Autodesk Fusion 360 part; units mm, degrees
(part 6 of 8)
  spline S1138 degree 3 poles (86.7419, -11.2934) (84.8369, -11.1346) (82.5615, -11.2934) (81.6884, -11.2934) knots 0 0 0 0 1 1 1 1
  spline S1139 degree 3 poles (81.6884, -11.2934) (80.7359, -11.2934) (80.5771, -11.0817) (80.3125, -10.6584) knots 0 0 0 0 1 1 1 1
  line L266 (80.3125, -10.6584) -> (72.6925, 1.486)
  line L267 (72.6925, 1.486) -> (72.6925, -8.9121)
  spline S1140 degree 3 poles (72.6925, -8.9121) (72.6925, -10.0498) (74.28, -9.9705) (74.28, -10.3938) knots 0 0 0 0 1 1 1 1
  spline S1141 degree 3 poles (74.28, -10.3938) (74.28, -10.7113) (73.989, -11.2934) (73.7773, -11.2669) knots 0 0 0 0 1 1 1 1
  spline S1142 degree 3 poles (73.7773, -11.2669) (73.3805, -11.214) (72.6132, -11.1902) (71.8459, -11.1902) knots 0 0 0 0 1 1 1 1
  spline S1143 degree 3 poles (71.8459, -11.1902) (71.0786, -11.1902) (70.2848, -11.214) (69.888, -11.2669) knots 0 0 0 0 1 1 1 1
  spline S1144 degree 3 poles (69.888, -11.2669) (69.6763, -11.2934) (69.4117, -10.7113) (69.4117, -10.3938) knots 0 0 0 0 1 1 1 1
  spline S1145 degree 3 poles (69.4117, -10.3938) (69.4117, -9.9705) (70.7082, -10.0498) (70.7082, -8.9121) knots 0 0 0 0 1 1 1 1
  spline S1146 degree 3 poles (250.4624, -9.4413) (247.4194, -9.4413) (245.779, -7.0865) (245.779, -2.4034) knots -1 -1 -1 -1 0 0 0 0
  spline S1147 degree 3 poles (252.1822, -8.8328) (252.1822, -9.4942) (251.7853, -9.4413) (250.4624, -9.4413) knots -1 -1 -1 -1 0 0 0 0
  line L268 (252.1822, -8.8328) -> (252.1822, 4.026)
  spline S1148 degree 3 poles (250.4357, 4.6345) (250.8328, 4.6345) (252.1822, 4.6875) (252.1822, 4.026) knots -1 -1 -1 -1 0 0 0 0
  spline S1149 degree 3 poles (245.779, -2.4034) (245.779, 2.2797) (247.4194, 4.6345) (250.4357, 4.6345) knots -1 -1 -1 -1 0 0 0 0
  spline S1150 degree 3 poles (239.9579, -2.3769) (239.9579, 2.9677) (243.6621, 6.5131) (249.245, 6.5131) knots 0 0 0 0 1 1 1 1
  spline S1151 degree 3 poles (249.245, 6.5131) (252.0234, 6.4866) (253.1082, 6.4337) (254.9606, 6.4337) knots 0 0 0 0 1 1 1 1
  spline S1152 degree 3 poles (254.9606, 6.4337) (256.1247, 6.4337) (257.4212, 6.4602) (258.4795, 6.5131) knots 0 0 0 0 1 1 1 1
  spline S1153 degree 3 poles (258.4795, 6.5131) (258.6912, 6.5131) (258.9558, 5.9575) (258.9558, 5.64) knots 0 0 0 0 1 1 1 1
  spline S1154 degree 3 poles (258.9558, 5.64) (258.9558, 5.2166) (257.527, 5.296) (257.527, 4.1583) knots 0 0 0 0 1 1 1 1
  line L269 (257.527, 4.1583) -> (257.527, -8.965)
  spline S1155 degree 3 poles (257.527, -8.965) (257.527, -10.0763) (258.9825, -9.9969) (258.9825, -10.4203) knots 0 0 0 0 1 1 1 1
  spline S1156 degree 3 poles (258.9825, -10.4203) (258.9825, -10.7378) (258.6912, -11.3225) (258.4795, -11.2934) knots 0 0 0 0 1 1 1 1
  spline S1157 degree 3 poles (258.4795, -11.2934) (257.4212, -11.2405) (256.1512, -11.214) (254.9606, -11.214) knots 0 0 0 0 1 1 1 1
  spline S1158 degree 3 poles (254.9606, -11.214) (253.1082, -11.214) (252.0234, -11.2934) (249.245, -11.2934) knots 0 0 0 0 1 1 1 1
  spline S1159 degree 3 poles (249.245, -11.2934) (243.6885, -11.2934) (239.9579, -7.7215) (239.9579, -2.3769) knots 0 0 0 0 1 1 1 1
  line L270 (70.7082, 2.0681) -> (70.7082, -8.9121)
  line L271 (70.7082, -8.9121) -> (70.7082, 2.0681)
  spline S1160 degree 3 poles (72.6925, -8.9121) (72.6925, -10.0498) (74.28, -9.9705) (74.28, -10.3938) knots 0 0 0 0 1 1 1 1
  spline S1161 degree 3 poles (74.28, -10.3938) (74.28, -9.9705) (72.6925, -10.0498) (72.6925, -8.9121) knots -1 -1 -1 -1 0 0 0 0
  spline S1162 degree 3 poles (239.9579, -2.3769) (239.9579, 2.9677) (243.6621, 6.5131) (249.245, 6.5131) knots 0 0 0 0 1 1 1 1
  spline S1163 degree 3 poles (249.245, 6.5131) (243.6621, 6.5131) (239.9579, 2.9677) (239.9579, -2.3769) knots -1 -1 -1 -1 0 0 0 0
  line L272 (83.9373, -6.2928) -> (76.2909, 5.9045)
  line L273 (76.2909, 5.9045) -> (83.9373, -6.2928)
  spline S1164 degree 3 poles (-114.9509, -10.3938) (-114.9509, -9.9705) (-113.7604, -9.9972) (-113.3886, -8.9388) knots 0 0 0 0 1 1 1 1
  spline S1165 degree 3 poles (-113.3886, -8.9388) (-113.7604, -9.9972) (-114.9509, -9.9705) (-114.9509, -10.3938) knots -1 -1 -1 -1 0 0 0 0
  line L274 (257.527, -8.965) -> (257.527, 4.1583)
  line L275 (257.527, 4.1583) -> (257.527, -8.965)
  line L276 (72.6925, -8.9121) -> (72.6925, 1.486)
  line L277 (72.6925, 1.486) -> (72.6925, -8.9121)
  spline S1166 degree 3 poles (254.9606, 6.4337) (256.1247, 6.4337) (257.4212, 6.4602) (258.4795, 6.5131) knots 0 0 0 0 1 1 1 1
  spline S1167 degree 3 poles (258.4795, 6.5131) (257.4212, 6.4602) (256.1247, 6.4337) (254.9606, 6.4337) knots -1 -1 -1 -1 0 0 0 0
  spline S1168 degree 3 poles (-91.5045, -10.3938) (-91.5045, -9.9705) (-89.8408, -9.9972) (-90.2088, -8.9388) knots 0 0 0 0 1 1 1 1
  spline S1169 degree 3 poles (-90.2088, -8.9388) (-89.8408, -9.9972) (-91.5045, -9.9705) (-91.5045, -10.3938) knots -1 -1 -1 -1 0 0 0 0
  line L278 (83.9373, 4.1583) -> (83.9373, -6.2928)
  line L279 (83.9373, -6.2928) -> (83.9373, 4.1583)
  spline S1170 degree 3 poles (258.9558, 5.64) (258.9558, 5.2166) (257.527, 5.296) (257.527, 4.1583) knots 0 0 0 0 1 1 1 1
  spline S1171 degree 3 poles (257.527, 4.1583) (257.527, 5.296) (258.9558, 5.2166) (258.9558, 5.64) knots -1 -1 -1 -1 0 0 0 0
  line L280 (72.6925, 1.486) -> (80.3125, -10.6584)
  line L281 (80.3125, -10.6584) -> (72.6925, 1.486)
  spline S1172 degree 3 poles (249.245, -11.2934) (243.6885, -11.2934) (239.9579, -7.7215) (239.9579, -2.3769) knots 0 0 0 0 1 1 1 1
  spline S1173 degree 3 poles (239.9579, -2.3769) (239.9579, -7.7215) (243.6885, -11.2934) (249.245, -11.2934) knots -1 -1 -1 -1 0 0 0 0
  spline S1174 degree 3 poles (120.1059, -10.4203) (120.1059, -10.0234) (121.5611, -10.1028) (121.5611, -8.965) knots 0 0 0 0 1 1 1 1
  line L282 (121.5611, -8.965) -> (121.5611, 3.7085)
  spline S1175 degree 3 poles (121.5611, 3.7085) (121.5611, 4.3964) (121.27, 4.5552) (119.6296, 4.5552) knots 0 0 0 0 1 1 1 1
  spline S1176 degree 3 poles (119.6296, 4.5552) (115.7667, 4.5552) (114.7348, 1.486) (114.2321, 1.486) knots 0 0 0 0 1 1 1 1
  spline S1177 degree 3 poles (114.2321, 1.486) (113.9146, 1.486) (113.3325, 1.7506) (113.3325, 1.9622) knots 0 0 0 0 1 1 1 1
  spline S1178 degree 3 poles (113.3325, 1.9622) (113.3325, 2.1739) (114.0469, 5.3489) (114.1527, 5.7458) knots 0 0 0 0 1 1 1 1
  spline S1179 degree 3 poles (114.1527, 5.7458) (114.338, 6.3543) (114.5496, 6.5395) (115.1052, 6.5131) knots 0 0 0 0 1 1 1 1
  spline S1180 degree 3 poles (115.1052, 6.5131) (116.9573, 6.4602) (119.2063, 6.4337) (121.4552, 6.4337) knots 0 0 0 0 1 1 1 1
  spline S1181 degree 3 poles (121.4552, 6.4337) (123.7307, 6.4337) (125.9796, 6.4602) (127.8317, 6.5131) knots 0 0 0 0 1 1 1 1
  spline S1182 degree 3 poles (127.8317, 6.5131) (128.0698, 6.5131) (128.3344, 5.9575) (128.3344, 5.64) knots 0 0 0 0 1 1 1 1
  spline S1183 degree 3 poles (128.3344, 5.64) (128.3344, 5.2166) (126.9057, 5.296) (126.9057, 4.1847) knots 0 0 0 0 1 1 1 1
  line L283 (126.9057, 4.1847) -> (126.9057, -8.965)
  spline S1184 degree 3 poles (126.9057, -8.965) (126.9057, -10.1028) (128.3344, -9.9969) (128.3344, -10.4203) knots 0 0 0 0 1 1 1 1
  spline S1185 degree 3 poles (128.3344, -10.4203) (128.3344, -10.7378) (128.0698, -11.3225) (127.8317, -11.2934) knots 0 0 0 0 1 1 1 1
  spline S1186 degree 3 poles (127.8317, -11.2934) (126.7734, -11.2405) (125.5034, -11.214) (124.2069, -11.214) knots 0 0 0 0 1 1 1 1
  spline S1187 degree 3 poles (124.2069, -11.214) (122.9369, -11.214) (121.6405, -11.2405) (120.6086, -11.2934) knots 0 0 0 0 1 1 1 1
  spline S1188 degree 3 poles (120.6086, -11.2934) (120.3969, -11.3225) (120.1059, -10.7378) (120.1059, -10.4203) knots 0 0 0 0 1 1 1 1
  spline S1189 degree 3 poles (-125.2401, 5.64) (-125.2401, 5.2164) (-127.0384, 5.1106) (-126.4299, 4.1584) knots 0 0 0 0 1 1 1 1
  spline S1190 degree 3 poles (-126.4299, 4.1584) (-127.0384, 5.1106) (-125.2401, 5.2164) (-125.2401, 5.64) knots -1 -1 -1 -1 0 0 0 0
  spline S1191 degree 3 poles (120.1059, -10.4203) (120.1059, -10.0234) (121.5611, -10.1028) (121.5611, -8.965) knots 0 0 0 0 1 1 1 1
  spline S1192 degree 3 poles (121.5611, -8.965) (121.5611, -10.1028) (120.1059, -10.0234) (120.1059, -10.4203) knots -1 -1 -1 -1 0 0 0 0
  spline S1193 degree 3 poles (121.5611, -8.965) (121.5611, -10.1028) (120.1059, -10.0234) (120.1059, -10.4203) knots -1 -1 -1 -1 0 0 0 0
  spline S1194 degree 3 poles (120.1059, -10.4203) (120.1059, -10.7378) (120.3969, -11.3225) (120.6086, -11.2934) knots -1 -1 -1 -1 0 0 0 0
  spline S1195 degree 3 poles (120.6086, -11.2934) (121.6405, -11.2405) (122.9369, -11.214) (124.2069, -11.214) knots -1 -1 -1 -1 0 0 0 0
  spline S1196 degree 3 poles (124.2069, -11.214) (125.5034, -11.214) (126.7734, -11.2405) (127.8317, -11.2934) knots -1 -1 -1 -1 0 0 0 0
  spline S1197 degree 3 poles (127.8317, -11.2934) (128.0698, -11.3225) (128.3344, -10.7378) (128.3344, -10.4203) knots -1 -1 -1 -1 0 0 0 0
  spline S1198 degree 3 poles (128.3344, -10.4203) (128.3344, -9.9969) (126.9057, -10.1028) (126.9057, -8.965) knots -1 -1 -1 -1 0 0 0 0
  line L284 (126.9057, -8.965) -> (126.9057, 4.1847)
  spline S1199 degree 3 poles (126.9057, 4.1847) (126.9057, 5.296) (128.3344, 5.2166) (128.3344, 5.64) knots -1 -1 -1 -1 0 0 0 0
  spline S1200 degree 3 poles (128.3344, 5.64) (128.3344, 5.9575) (128.0698, 6.5131) (127.8317, 6.5131) knots -1 -1 -1 -1 0 0 0 0
  spline S1201 degree 3 poles (127.8317, 6.5131) (125.9796, 6.4602) (123.7307, 6.4337) (121.4552, 6.4337) knots -1 -1 -1 -1 0 0 0 0
  spline S1202 degree 3 poles (121.4552, 6.4337) (119.2063, 6.4337) (116.9573, 6.4602) (115.1052, 6.5131) knots -1 -1 -1 -1 0 0 0 0
  spline S1203 degree 3 poles (115.1052, 6.5131) (114.5496, 6.5395) (114.338, 6.3543) (114.1527, 5.7458) knots -1 -1 -1 -1 0 0 0 0
  spline S1204 degree 3 poles (114.1527, 5.7458) (114.0469, 5.3489) (113.3325, 2.1739) (113.3325, 1.9622) knots -1 -1 -1 -1 0 0 0 0
  spline S1205 degree 3 poles (113.3325, 1.9622) (113.3325, 1.7506) (113.9146, 1.486) (114.2321, 1.486) knots -1 -1 -1 -1 0 0 0 0
  spline S1206 degree 3 poles (114.2321, 1.486) (114.7348, 1.486) (115.7667, 4.5552) (119.6296, 4.5552) knots -1 -1 -1 -1 0 0 0 0
  spline S1207 degree 3 poles (119.6296, 4.5552) (121.27, 4.5552) (121.5611, 4.3964) (121.5611, 3.7085) knots -1 -1 -1 -1 0 0 0 0
  line L285 (121.5611, 3.7085) -> (121.5611, -8.965)
  spline S1208 degree 3 poles (250.4624, -9.4413) (247.4194, -9.4413) (245.779, -7.0865) (245.779, -2.4034) knots -1 -1 -1 -1 0 0 0 0
  spline S1209 degree 3 poles (250.4624, -9.4413) (247.4194, -9.4413) (245.779, -7.0865) (245.779, -2.4034) knots -1 -1 -1 -1 0 0 0 0
  spline S1210 degree 3 poles (250.4624, -9.4413) (247.4194, -9.4413) (245.779, -7.0865) (245.779, -2.4034) knots -1 -1 -1 -1 0 0 0 0
  spline S1211 degree 3 poles (245.779, -2.4034) (245.779, 2.2797) (247.4194, 4.6345) (250.4357, 4.6345) knots -1 -1 -1 -1 0 0 0 0
  spline S1212 degree 3 poles (250.4357, 4.6345) (250.8328, 4.6345) (252.1822, 4.6875) (252.1822, 4.026) knots -1 -1 -1 -1 0 0 0 0
  line L286 (252.1822, 4.026) -> (252.1822, -8.8328)
  spline S1213 degree 3 poles (252.1822, -8.8328) (252.1822, -9.4942) (251.7853, -9.4413) (250.4624, -9.4413) knots -1 -1 -1 -1 0 0 0 0
  spline S1214 degree 3 poles (249.245, 6.5131) (243.6621, 6.5131) (239.9579, 2.9677) (239.9579, -2.3769) knots -1 -1 -1 -1 0 0 0 0
  spline S1215 degree 3 poles (239.9579, -2.3769) (239.9579, -7.7215) (243.6885, -11.2934) (249.245, -11.2934) knots -1 -1 -1 -1 0 0 0 0
  spline S1216 degree 3 poles (249.245, -11.2934) (252.0234, -11.2934) (253.1082, -11.214) (254.9606, -11.214) knots -1 -1 -1 -1 0 0 0 0
  spline S1217 degree 3 poles (254.9606, -11.214) (256.1512, -11.214) (257.4212, -11.2405) (258.4795, -11.2934) knots -1 -1 -1 -1 0 0 0 0
  spline S1218 degree 3 poles (258.4795, -11.2934) (258.6912, -11.3225) (258.9825, -10.7378) (258.9825, -10.4203) knots -1 -1 -1 -1 0 0 0 0
  spline S1219 degree 3 poles (258.9825, -10.4203) (258.9825, -9.9969) (257.527, -10.0763) (257.527, -8.965) knots -1 -1 -1 -1 0 0 0 0
  line L287 (257.527, -8.965) -> (257.527, 4.1583)
  spline S1220 degree 3 poles (257.527, 4.1583) (257.527, 5.296) (258.9558, 5.2166) (258.9558, 5.64) knots -1 -1 -1 -1 0 0 0 0
  spline S1221 degree 3 poles (258.9558, 5.64) (258.9558, 5.9575) (258.6912, 6.5131) (258.4795, 6.5131) knots -1 -1 -1 -1 0 0 0 0
  spline S1222 degree 3 poles (258.4795, 6.5131) (257.4212, 6.4602) (256.1247, 6.4337) (254.9606, 6.4337) knots -1 -1 -1 -1 0 0 0 0
  spline S1223 degree 3 poles (254.9606, 6.4337) (253.1082, 6.4337) (252.0234, 6.4866) (249.245, 6.5131) knots -1 -1 -1 -1 0 0 0 0
  spline S1224 degree 3 poles (263.4264, -11.0288) (262.765, -11.0288) (262.5533, -11.2934) (262.1297, -11.2934) knots 0 0 0 0 1 1 1 1
  spline S1225 degree 3 poles (262.1297, -11.2934) (262.5533, -11.2934) (262.765, -11.0288) (263.4264, -11.0288) knots -1 -1 -1 -1 0 0 0 0
  spline S1226 degree 3 poles (276.4447, -2.3769) (276.4447, -7.748) (272.6876, -11.558) (267.4219, -11.558) knots 0 0 0 0 1 1 1 1
  spline S1227 degree 3 poles (267.4219, -11.558) (272.6876, -11.558) (276.4447, -7.748) (276.4447, -2.3769) knots -1 -1 -1 -1 0 0 0 0
  spline S1228 degree 3 poles (266.6546, -9.653) (269.1417, -9.653) (270.6236, -7.2717) (270.6236, -3.303) knots 0 0 0 0 1 1 1 1
  spline S1229 degree 3 poles (270.6236, -3.303) (270.6236, -7.2717) (269.1417, -9.653) (266.6546, -9.653) knots -1 -1 -1 -1 0 0 0 0
  spline S1230 degree 3 poles (-167.8359, 5.746) (-167.6766, 6.3543) (-167.4397, 6.5397) (-166.9127, 6.5132) knots 0 0 0 0 1 1 1 1
  spline S1231 degree 3 poles (-166.9127, 6.5132) (-167.4397, 6.5397) (-167.6766, 6.3543) (-167.8359, 5.746) knots -1 -1 -1 -1 0 0 0 0
  spline S1232 degree 3 poles (-153.918, -6.1339) (-153.5994, -6.1339) (-153.0438, -6.4252) (-153.0438, -6.6368) knots 0 0 0 0 1 1 1 1
  spline S1233 degree 3 poles (-153.0438, -6.6368) (-153.0438, -6.4252) (-153.5994, -6.1339) (-153.918, -6.1339) knots -1 -1 -1 -1 0 0 0 0
  spline S1234 degree 3 poles (-154.6329, -11.2934) (-158.334, -11.2138) (-163.9224, -11.1901) (-167.6235, -11.2934) knots 0 0 0 0 1 1 1 1
  spline S1235 degree 3 poles (-167.6235, -11.2934) (-163.9224, -11.1901) (-158.334, -11.2138) (-154.6329, -11.2934) knots -1 -1 -1 -1 0 0 0 0
  spline S1236 degree 3 poles (68.1959, -2.3768) (68.1959, -7.8007) (64.3845, -11.5577) (58.909, -11.5577) knots 0 0 0 0 1 1 1 1
  spline S1237 degree 3 poles (58.909, -11.5577) (64.3845, -11.5577) (68.1959, -7.8007) (68.1959, -2.3768) knots -1 -1 -1 -1 0 0 0 0
  spline S1238 degree 3 poles (49.6221, -2.3768) (49.6221, 3.0471) (53.406, 6.7777) (58.909, 6.7777) knots 0 0 0 0 1 1 1 1
  spline S1239 degree 3 poles (58.909, 6.7777) (53.406, 6.7777) (49.6221, 3.0471) (49.6221, -2.3768) knots -1 -1 -1 -1 0 0 0 0
  spline S1240 degree 3 poles (-120.4768, 5.6133) (-120.4768, 5.9311) (-120.1048, 6.5396) (-119.8955, 6.5132) knots 0 0 0 0 1 1 1 1
  spline S1241 degree 3 poles (-119.8955, 6.5132) (-120.1048, 6.5396) (-120.4768, 5.9311) (-120.4768, 5.6133) knots -1 -1 -1 -1 0 0 0 0
  spline S1242 degree 3 poles (55.4435, -2.3768) (55.4435, 2.5179) (56.5282, 4.9256) (58.909, 4.9256) knots -1 -1 -1 -1 0 0 0 0
  spline S1243 degree 3 poles (58.909, -9.7058) (56.5529, -9.7058) (55.4435, -7.3509) (55.4435, -2.3768) knots -1 -1 -1 -1 0 0 0 0
  spline S1244 degree 3 poles (62.3744, -2.3768) (62.3744, -7.2715) (61.2897, -9.7058) (58.909, -9.7058) knots -1 -1 -1 -1 0 0 0 0
  spline S1245 degree 3 poles (58.909, 4.9256) (61.2897, 4.9256) (62.3744, 2.5179) (62.3744, -2.3768) knots -1 -1 -1 -1 0 0 0 0
  spline S1246 degree 3 poles (68.1959, -2.3768) (68.1959, -7.8007) (64.3845, -11.5577) (58.909, -11.5577) knots 0 0 0 0 1 1 1 1
  spline S1247 degree 3 poles (58.909, -11.5577) (53.4307, -11.5577) (49.6221, -7.8007) (49.6221, -2.3768) knots 0 0 0 0 1 1 1 1
  spline S1248 degree 3 poles (49.6221, -2.3768) (49.6221, 3.0471) (53.406, 6.7777) (58.909, 6.7777) knots 0 0 0 0 1 1 1 1
  spline S1249 degree 3 poles (58.909, 6.7777) (64.4119, 6.7777) (68.1959, 3.0471) (68.1959, -2.3768) knots 0 0 0 0 1 1 1 1
  spline S1250 degree 3 poles (55.4435, -2.3768) (55.4435, 2.5179) (56.5282, 4.9256) (58.909, 4.9256) knots -1 -1 -1 -1 0 0 0 0
  spline S1251 degree 3 poles (58.909, 4.9256) (61.2897, 4.9256) (62.3744, 2.5179) (62.3744, -2.3768) knots -1 -1 -1 -1 0 0 0 0
  spline S1252 degree 3 poles (62.3744, -2.3768) (62.3744, -7.2715) (61.2897, -9.7058) (58.909, -9.7058) knots -1 -1 -1 -1 0 0 0 0
  spline S1253 degree 3 poles (58.909, -9.7058) (56.5529, -9.7058) (55.4435, -7.3509) (55.4435, -2.3768) knots -1 -1 -1 -1 0 0 0 0
  spline S1254 degree 3 poles (58.909, -11.5577) (64.3845, -11.5577) (68.1959, -7.8007) (68.1959, -2.3768) knots -1 -1 -1 -1 0 0 0 0
  spline S1255 degree 3 poles (68.1959, -2.3768) (68.1959, 3.0471) (64.4119, 6.7777) (58.909, 6.7777) knots -1 -1 -1 -1 0 0 0 0
  spline S1256 degree 3 poles (58.909, 6.7777) (53.406, 6.7777) (49.6221, 3.0471) (49.6221, -2.3768) knots -1 -1 -1 -1 0 0 0 0
  spline S1257 degree 3 poles (49.6221, -2.3768) (49.6221, -7.8007) (53.4307, -11.5577) (58.909, -11.5577) knots -1 -1 -1 -1 0 0 0 0
  spline S1258 degree 3 poles (58.909, -9.7058) (56.5529, -9.7058) (55.4435, -7.3509) (55.4435, -2.3768) knots -1 -1 -1 -1 0 0 0 0
  spline S1259 degree 3 poles (58.909, -9.7058) (56.5529, -9.7058) (55.4435, -7.3509) (55.4435, -2.3768) knots -1 -1 -1 -1 0 0 0 0
  spline S1260 degree 3 poles (58.909, -11.5577) (53.4307, -11.5577) (49.6221, -7.8007) (49.6221, -2.3768) knots 0 0 0 0 1 1 1 1
  spline S1261 degree 3 poles (49.6221, -2.3768) (49.6221, -7.8007) (53.4307, -11.5577) (58.909, -11.5577) knots -1 -1 -1 -1 0 0 0 0
  spline S1262 degree 3 poles (-159.9516, 3.7083) (-159.6044, 4.2905) (-160.2417, 4.5552) (-161.5939, 4.5552) knots 0 0 0 0 1 1 1 1
  spline S1263 degree 3 poles (-161.5939, 4.5552) (-160.2417, 4.5552) (-159.6044, 4.2905) (-159.9516, 3.7083) knots -1 -1 -1 -1 0 0 0 0
  line L288 (151.9352, 6.2485) -> (151.9352, -8.9386)
  spline S1264 degree 3 poles (151.9352, -8.9386) (151.9352, -10.0763) (150.48, -9.9969) (150.48, -10.3938) knots -1 -1 -1 -1 0 0 0 0
  spline S1265 degree 3 poles (150.48, -10.3938) (150.48, -10.7113) (150.7684, -11.2934) (150.9827, -11.2934) knots -1 -1 -1 -1 0 0 0 0
  spline S1266 degree 3 poles (150.9827, -11.2934) (152.012, -11.2405) (153.3111, -11.214) (154.6075, -11.214) knots -1 -1 -1 -1 0 0 0 0
  spline S1267 degree 3 poles (154.6075, -11.214) (155.8775, -11.214) (157.174, -11.2405) (158.2323, -11.2934) knots -1 -1 -1 -1 0 0 0 0
  spline S1268 degree 3 poles (158.2323, -11.2934) (158.444, -11.2934) (158.7086, -10.7113) (158.7086, -10.3938) knots -1 -1 -1 -1 0 0 0 0
  spline S1269 degree 3 poles (158.7086, -10.3938) (158.7086, -9.9969) (157.2798, -10.0763) (157.2798, -8.9386) knots -1 -1 -1 -1 0 0 0 0
  line L289 (157.2798, -8.9386) -> (157.2798, 6.4866)
  spline S1270 degree 3 poles (157.2798, 6.4866) (157.2798, 9.6881) (158.4175, 10.6141) (161.0634, 10.6141) knots -1 -1 -1 -1 0 0 0 0
  spline S1271 degree 3 poles (161.0634, 10.6141) (161.3015, 10.6141) (161.7248, 11.5931) (161.5661, 11.7518) knots -1 -1 -1 -1 0 0 0 0
  spline S1272 degree 3 poles (161.5661, 11.7518) (161.2221, 12.0958) (159.7669, 12.5985) (157.7825, 12.5985) knots -1 -1 -1 -1 0 0 0 0
  spline S1273 degree 3 poles (157.7825, 12.5985) (153.8932, 12.5985) (151.9352, 10.5612) (151.9352, 6.2485) knots -1 -1 -1 -1 0 0 0 0
  line L290 (-84.4965, -8.9388) -> (-89.9196, 6.5129)
  line L291 (-89.9196, 6.5129) -> (-94.7607, 6.5129)
  spline S1274 degree 3 poles (-94.7607, 6.5129) (-95.2114, 3.9993) (-97.7765, -0.8688) (-99.0459, -5.0229) knots -1 -1 -1 -1 0 0 0 0
  line L292 (-99.0459, -5.0229) -> (-103.0944, 6.5129)
  spline S1275 degree 3 poles (-103.0944, 6.5129) (-104.0221, 6.46) (-104.7619, 6.4337) (-105.5281, 6.4337) knots -1 -1 -1 -1 0 0 0 0
  spline S1276 degree 3 poles (-105.5281, 6.4337) (-106.2717, 6.4337) (-107.0378, 6.46) (-107.9354, 6.5129) knots -1 -1 -1 -1 0 0 0 0
  line L293 (-107.9354, 6.5129) -> (-113.3886, -8.9388)
  spline S1277 degree 3 poles (-113.3886, -8.9388) (-113.7604, -9.9972) (-114.9509, -9.9705) (-114.9509, -10.3938) knots -1 -1 -1 -1 0 0 0 0
  spline S1278 degree 3 poles (-114.9509, -10.3938) (-114.9509, -10.7115) (-114.688, -11.2936) (-114.4439, -11.267) knots -1 -1 -1 -1 0 0 0 0
  spline S1279 degree 3 poles (-114.4439, -11.267) (-114.0496, -11.214) (-113.2534, -11.1903) (-112.4609, -11.1903) knots -1 -1 -1 -1 0 0 0 0
  spline S1280 degree 3 poles (-112.4609, -11.1903) (-111.6685, -11.1903) (-110.8723, -11.214) (-110.478, -11.267) knots -1 -1 -1 -1 0 0 0 0
  spline S1281 degree 3 poles (-110.478, -11.267) (-110.2639, -11.2936) (-109.9747, -10.7115) (-109.9747, -10.3938) knots -1 -1 -1 -1 0 0 0 0
  spline S1282 degree 3 poles (-109.9747, -10.3938) (-109.9747, -9.9705) (-111.6422, -9.9972) (-111.2704, -8.9122) knots -1 -1 -1 -1 0 0 0 0
  line L294 (-111.2704, -8.9122) -> (-107.327, 2.4384)
  line L295 (-107.327, 2.4384) -> (-103.3873, -8.9122)
  spline S1283 degree 3 poles (-103.3873, -8.9122) (-103.0155, -9.9972) (-104.7093, -9.9705) (-104.7093, -10.3938) knots -1 -1 -1 -1 0 0 0 0
  spline S1284 degree 3 poles (-104.7093, -10.3938) (-104.7093, -10.7115) (-104.4163, -11.267) (-104.206, -11.267) knots -1 -1 -1 -1 0 0 0 0
  spline S1285 degree 3 poles (-104.206, -11.267) (-103.1733, -11.214) (-101.7987, -11.1903) (-100.3978, -11.1903) knots -1 -1 -1 -1 0 0 0 0
  spline S1286 degree 3 poles (-100.3978, -11.1903) (-99.0195, -11.1903) (-97.645, -11.214) (-96.5859, -11.267) knots -1 -1 -1 -1 0 0 0 0
  spline S1287 degree 3 poles (-96.5859, -11.267) (-96.3755, -11.267) (-96.1089, -10.7115) (-96.1089, -10.3938) knots -1 -1 -1 -1 0 0 0 0
  spline S1288 degree 3 poles (-96.1089, -10.3938) (-96.1089, -9.9705) (-97.2994, -9.9972) (-97.6712, -8.9388) knots -1 -1 -1 -1 0 0 0 0
  spline S1289 degree 3 poles (-97.6712, -8.9388) (-98.1219, -7.0866) (-95.3165, -1.2924) (-94.0996, 2.2533) knots -1 -1 -1 -1 0 0 0 0
  line L296 (-94.0996, 2.2533) -> (-90.2088, -8.9388)
  spline S1290 degree 3 poles (-90.2088, -8.9388) (-89.8408, -9.9972) (-91.5045, -9.9705) (-91.5045, -10.3938) knots -1 -1 -1 -1 0 0 0 0
  spline S1291 degree 3 poles (-91.5045, -10.3938) (-91.5045, -10.7115) (-91.2416, -11.267) (-91.0313, -11.267) knots -1 -1 -1 -1 0 0 0 0
  spline S1292 degree 3 poles (-91.0313, -11.267) (-89.9722, -11.214) (-88.5939, -11.1903) (-87.2194, -11.1903) knots -1 -1 -1 -1 0 0 0 0
  spline S1293 degree 3 poles (-87.2194, -11.1903) (-85.8448, -11.1903) (-84.4664, -11.214) (-83.4111, -11.267) knots -1 -1 -1 -1 0 0 0 0
  spline S1294 degree 3 poles (-83.4111, -11.267) (-83.1971, -11.267) (-82.9079, -10.7115) (-82.9079, -10.3938) knots -1 -1 -1 -1 0 0 0 0
  spline S1295 degree 3 poles (-82.9079, -10.3938) (-82.9079, -9.9705) (-84.1247, -9.9972) (-84.4965, -8.9388) knots -1 -1 -1 -1 0 0 0 0
  spline S1296 degree 3 poles (158.7086, -10.3938) (158.7086, -10.7113) (158.444, -11.2934) (158.2323, -11.2934) knots 0 0 0 0 1 1 1 1
  spline S1297 degree 3 poles (158.2323, -11.2934) (158.444, -11.2934) (158.7086, -10.7113) (158.7086, -10.3938) knots -1 -1 -1 -1 0 0 0 0
  spline S1298 degree 3 poles (-153.2807, 6.5132) (-153.0438, 6.5132) (-152.7783, 5.9576) (-152.7783, 5.6398) knots 0 0 0 0 1 1 1 1
  spline S1299 degree 3 poles (-152.7783, 5.6398) (-152.7783, 5.9576) (-153.0438, 6.5132) (-153.2807, 6.5132) knots -1 -1 -1 -1 0 0 0 0
  spline S1300 degree 3 poles (82.3498, 5.6135) (82.3498, 5.931) (82.6409, 6.5395) (82.8525, 6.5131) knots 0 0 0 0 1 1 1 1
  spline S1301 degree 3 poles (82.8525, 6.5131) (82.6409, 6.5395) (82.3498, 5.931) (82.3498, 5.6135) knots -1 -1 -1 -1 0 0 0 0
  spline S1302 degree 3 poles (86.7419, -11.2934) (84.8369, -11.1346) (82.5615, -11.2934) (81.6884, -11.2934) knots 0 0 0 0 1 1 1 1
  spline S1303 degree 3 poles (81.6884, -11.2934) (82.5615, -11.2934) (84.8369, -11.1346) (86.7419, -11.2934) knots -1 -1 -1 -1 0 0 0 0
  spline S1304 degree 3 poles (226.6509, 0.507) (226.6509, 0.7187) (227.233, 1.0097) (227.5505, 1.0097) knots 0 0 0 0 1 1 1 1
  spline S1305 degree 3 poles (227.5505, 1.0097) (227.233, 1.0097) (226.6509, 0.7187) (226.6509, 0.507) knots -1 -1 -1 -1 0 0 0 0
  spline S1306 degree 3 poles (237.5515, -8.9386) (237.5515, -10.0763) (238.9803, -9.9969) (238.9803, -10.3938) knots 0 0 0 0 1 1 1 1
  spline S1307 degree 3 poles (238.9803, -10.3938) (238.9803, -9.9969) (237.5515, -10.0763) (237.5515, -8.9386) knots -1 -1 -1 -1 0 0 0 0
  spline S1308 degree 3 poles (227.5505, 1.0097) (228.3443, 1.0097) (228.1855, -1.7155) (230.3551, -1.7684) knots 0 0 0 0 1 1 1 1
  spline S1309 degree 3 poles (230.3551, -1.7684) (228.1855, -1.7155) (228.3443, 1.0097) (227.5505, 1.0097) knots -1 -1 -1 -1 0 0 0 0
  line L297 (237.5515, -8.9386) -> (237.5515, 4.1847)
  line L298 (237.5515, 4.1847) -> (237.5515, -8.9386)
  line L299 (232.2072, -1.8213) -> (230.3551, -1.7684)
  line L300 (230.3551, -1.7684) -> (232.2072, -1.8213)
  spline S1310 degree 3 poles (-82.9079, -10.3938) (-82.9079, -10.7115) (-83.1971, -11.267) (-83.4111, -11.267) knots 0 0 0 0 1 1 1 1
  spline S1311 degree 3 poles (-83.4111, -11.267) (-83.1971, -11.267) (-82.9079, -10.7115) (-82.9079, -10.3938) knots -1 -1 -1 -1 0 0 0 0
  spline S1312 degree 3 poles (154.6075, -11.214) (153.3111, -11.214) (152.012, -11.2405) (150.9827, -11.2934) knots 0 0 0 0 1 1 1 1
  spline S1313 degree 3 poles (150.9827, -11.2934) (152.012, -11.2405) (153.3111, -11.214) (154.6075, -11.214) knots -1 -1 -1 -1 0 0 0 0
  spline S1314 degree 3 poles (-134.0225, 6.5132) (-132.9915, 6.4601) (-131.4296, 6.4338) (-129.8948, 6.4338) knots 0 0 0 0 1 1 1 1
  spline S1315 degree 3 poles (-129.8948, 6.4338) (-131.4296, 6.4338) (-132.9915, 6.4601) (-134.0225, 6.5132) knots -1 -1 -1 -1 0 0 0 0
  spline S1316 degree 3 poles (121.4552, 6.4337) (123.7307, 6.4337) (125.9796, 6.4602) (127.8317, 6.5131) knots 0 0 0 0 1 1 1 1
  spline S1317 degree 3 poles (127.8317, 6.5131) (125.9796, 6.4602) (123.7307, 6.4337) (121.4552, 6.4337) knots -1 -1 -1 -1 0 0 0 0
  spline S1318 degree 3 poles (124.2069, -11.214) (122.9369, -11.214) (121.6405, -11.2405) (120.6086, -11.2934) knots 0 0 0 0 1 1 1 1
  spline S1319 degree 3 poles (120.6086, -11.2934) (121.6405, -11.2405) (122.9369, -11.214) (124.2069, -11.214) knots -1 -1 -1 -1 0 0 0 0
  spline S1320 degree 3 poles (120.6086, -11.2934) (120.3969, -11.3225) (120.1059, -10.7378) (120.1059, -10.4203) knots 0 0 0 0 1 1 1 1
  spline S1321 degree 3 poles (120.1059, -10.4203) (120.1059, -10.7378) (120.3969, -11.3225) (120.6086, -11.2934) knots -1 -1 -1 -1 0 0 0 0
  spline S1322 degree 3 poles (223.3172, 1.9622) (223.3172, 2.1739) (224.0316, 5.3489) (224.1374, 5.7458) knots 0 0 0 0 1 1 1 1
  spline S1323 degree 3 poles (224.1374, 5.7458) (224.0316, 5.3489) (223.3172, 2.1739) (223.3172, 1.9622) knots -1 -1 -1 -1 0 0 0 0
  spline S1324 degree 3 poles (-166.9127, 6.5132) (-165.0581, 6.4601) (-162.5703, 6.4339) (-160.1069, 6.4339) knots 0 0 0 0 1 1 1 1
  spline S1325 degree 3 poles (-160.1069, 6.4339) (-162.5703, 6.4339) (-165.0581, 6.4601) (-166.9127, 6.5132) knots -1 -1 -1 -1 0 0 0 0
  spline S1326 degree 3 poles (161.0634, 10.6141) (158.4175, 10.6141) (157.2798, 9.6881) (157.2798, 6.4866) knots 0 0 0 0 1 1 1 1
  spline S1327 degree 3 poles (157.2798, 6.4866) (157.2798, 9.6881) (158.4175, 10.6141) (161.0634, 10.6141) knots -1 -1 -1 -1 0 0 0 0
  spline S1328 degree 3 poles (-168.657, 1.9624) (-168.657, 2.174) (-167.9421, 5.3489) (-167.8359, 5.746) knots 0 0 0 0 1 1 1 1
  spline S1329 degree 3 poles (-167.8359, 5.746) (-167.9421, 5.3489) (-168.657, 2.174) (-168.657, 1.9624) knots -1 -1 -1 -1 0 0 0 0
  spline S1330 degree 3 poles (157.2798, -8.9386) (157.2798, -10.0763) (158.7086, -9.9969) (158.7086, -10.3938) knots 0 0 0 0 1 1 1 1
  spline S1331 degree 3 poles (158.7086, -10.3938) (158.7086, -9.9969) (157.2798, -10.0763) (157.2798, -8.9386) knots -1 -1 -1 -1 0 0 0 0
  spline S1332 degree 3 poles (-153.0438, -6.6368) (-153.0438, -6.8484) (-153.6525, -10.1292) (-153.7301, -10.5524) knots 0 0 0 0 1 1 1 1
  spline S1333 degree 3 poles (-153.7301, -10.5524) (-153.6525, -10.1292) (-153.0438, -6.8484) (-153.0438, -6.6368) knots -1 -1 -1 -1 0 0 0 0
  spline S1334 degree 3 poles (-114.4439, -11.267) (-114.688, -11.2936) (-114.9509, -10.7115) (-114.9509, -10.3938) knots 0 0 0 0 1 1 1 1
  spline S1335 degree 3 poles (-114.9509, -10.3938) (-114.9509, -10.7115) (-114.688, -11.2936) (-114.4439, -11.267) knots -1 -1 -1 -1 0 0 0 0
  spline S1336 degree 3 poles (83.9373, 4.1583) (83.9373, 5.296) (82.3498, 5.2166) (82.3498, 5.6135) knots 0 0 0 0 1 1 1 1
  spline S1337 degree 3 poles (82.3498, 5.6135) (82.3498, 5.2166) (83.9373, 5.296) (83.9373, 4.1583) knots -1 -1 -1 -1 0 0 0 0
  line L301 (-94.0996, 2.2533) -> (-90.2088, -8.9388)
  line L302 (-90.2088, -8.9388) -> (-94.0996, 2.2533)
  spline S1338 degree 3 poles (81.6884, -11.2934) (80.7359, -11.2934) (80.5771, -11.0817) (80.3125, -10.6584) knots 0 0 0 0 1 1 1 1
  spline S1339 degree 3 poles (80.3125, -10.6584) (80.5771, -11.0817) (80.7359, -11.2934) (81.6884, -11.2934) knots -1 -1 -1 -1 0 0 0 0
  spline S1340 degree 3 poles (-112.4609, -11.1903) (-113.2534, -11.1903) (-114.0496, -11.214) (-114.4439, -11.267) knots 0 0 0 0 1 1 1 1
  spline S1341 degree 3 poles (-114.4439, -11.267) (-114.0496, -11.214) (-113.2534, -11.1903) (-112.4609, -11.1903) knots -1 -1 -1 -1 0 0 0 0
  spline S1342 degree 3 poles (223.6347, -10.6848) (223.6347, -10.1028) (224.0316, -6.9807) (224.0316, -6.769) knots 0 0 0 0 1 1 1 1
  spline S1343 degree 3 poles (224.0316, -6.769) (224.0316, -6.9807) (223.6347, -10.1028) (223.6347, -10.6848) knots -1 -1 -1 -1 0 0 0 0
  spline S1344 degree 3 poles (227.5505, -6.5044) (227.233, -6.5044) (226.6509, -6.2134) (226.6509, -6.0017) knots 0 0 0 0 1 1 1 1
  spline S1345 degree 3 poles (226.6509, -6.0017) (226.6509, -6.2134) (227.233, -6.5044) (227.5505, -6.5044) knots -1 -1 -1 -1 0 0 0 0
  spline S1346 degree 3 poles (238.4778, -11.2934) (236.7313, -11.2405) (234.3236, -11.214) (231.8897, -11.214) knots 0 0 0 0 1 1 1 1
  spline S1347 degree 3 poles (231.8897, -11.214) (234.3236, -11.214) (236.7313, -11.2405) (238.4778, -11.2934) knots -1 -1 -1 -1 0 0 0 0
  spline S1348 degree 3 poles (226.6509, -6.0017) (226.7832, -3.8321) (226.7832, -1.6625) (226.6509, 0.507) knots 0 0 0 0 1 1 1 1
  spline S1349 degree 3 poles (226.6509, 0.507) (226.7832, -1.6625) (226.7832, -3.8321) (226.6509, -6.0017) knots -1 -1 -1 -1 0 0 0 0
  spline S1350 degree 3 poles (238.9803, -10.3938) (238.9803, -10.7113) (238.7157, -11.2934) (238.4778, -11.2934) knots 0 0 0 0 1 1 1 1
  spline S1351 degree 3 poles (238.4778, -11.2934) (238.7157, -11.2934) (238.9803, -10.7113) (238.9803, -10.3938) knots -1 -1 -1 -1 0 0 0 0
  spline S1352 degree 3 poles (265.5433, 3.7879) (263.8233, 3.7879) (262.4475, 3.0206) (260.8862, 1.2743) knots 0 0 0 0 1 1 1 1
  spline S1353 degree 3 poles (260.8862, 1.2743) (262.4475, 3.0206) (263.8233, 3.7879) (265.5433, 3.7879) knots -1 -1 -1 -1 0 0 0 0
  spline S1354 degree 3 poles (270.6236, -3.303) (270.6236, 1.195) (268.7186, 3.7879) (265.5433, 3.7879) knots 0 0 0 0 1 1 1 1
  spline S1355 degree 3 poles (265.5433, 3.7879) (263.8233, 3.7879) (262.4475, 3.0206) (260.8862, 1.2743) knots 0 0 0 0 1 1 1 1
  spline S1356 degree 3 poles (260.8862, 1.2743) (260.7277, 1.0891) (259.9339, 1.3272) (259.9339, 1.5389) knots 0 0 0 0 1 1 1 1
  spline S1357 degree 3 poles (259.9339, 1.5389) (259.9339, 2.412) (262.2093, 6.7777) (267.66, 6.7777) knots 0 0 0 0 1 1 1 1
  spline S1358 degree 3 poles (267.66, 6.7777) (272.767, 6.7777) (276.4447, 2.9412) (276.4447, -2.3769) knots 0 0 0 0 1 1 1 1
  spline S1359 degree 3 poles (276.4447, -2.3769) (276.4447, -7.748) (272.6876, -11.558) (267.4219, -11.558) knots 0 0 0 0 1 1 1 1
  spline S1360 degree 3 poles (267.4219, -11.558) (265.305, -11.558) (264.326, -11.0288) (263.4264, -11.0288) knots 0 0 0 0 1 1 1 1
  spline S1361 degree 3 poles (263.4264, -11.0288) (262.765, -11.0288) (262.5533, -11.2934) (262.1297, -11.2934) knots 0 0 0 0 1 1 1 1
  spline S1362 degree 3 poles (262.1297, -11.2934) (261.786, -11.2934) (261.5743, -10.9759) (261.442, -10.4732) knots 0 0 0 0 1 1 1 1
  spline S1363 degree 3 poles (261.442, -10.4732) (261.336, -10.0763) (260.7539, -6.7161) (260.7539, -6.5044) knots 0 0 0 0 1 1 1 1
  spline S1364 degree 3 poles (260.7539, -6.5044) (260.7539, -6.2928) (261.336, -5.7371) (261.6537, -5.7371) knots 0 0 0 0 1 1 1 1
  spline S1365 degree 3 poles (261.6537, -5.7371) (262.1297, -5.7371) (263.4529, -9.653) (266.6546, -9.653) knots 0 0 0 0 1 1 1 1
  spline S1366 degree 3 poles (266.6546, -9.653) (269.1417, -9.653) (270.6236, -7.2717) (270.6236, -3.303) knots 0 0 0 0 1 1 1 1
  spline S1367 degree 3 poles (270.6236, -3.303) (270.6236, 1.195) (268.7186, 3.7879) (265.5433, 3.7879) knots 0 0 0 0 1 1 1 1
  spline S1368 degree 3 poles (265.5433, 3.7879) (268.7186, 3.7879) (270.6236, 1.195) (270.6236, -3.303) knots -1 -1 -1 -1 0 0 0 0
  line L303 (157.2798, -8.9386) -> (157.2798, 6.4866)
  line L304 (157.2798, 6.4866) -> (157.2798, -8.9386)
  spline S1369 degree 3 poles (-168.126, -10.42) (-168.126, -10.0234) (-168.1791, -9.9175) (-167.599, -8.9649) knots 0 0 0 0 1 1 1 1
  spline S1370 degree 3 poles (-167.599, -8.9649) (-168.1791, -9.9175) (-168.126, -10.0234) (-168.126, -10.42) knots -1 -1 -1 -1 0 0 0 0
  spline S1371 degree 3 poles (150.9827, -11.2934) (150.7684, -11.2934) (150.48, -10.7113) (150.48, -10.3938) knots 0 0 0 0 1 1 1 1
  spline S1372 degree 3 poles (150.48, -10.3938) (150.48, -10.7113) (150.7684, -11.2934) (150.9827, -11.2934) knots -1 -1 -1 -1 0 0 0 0
  line L305 (-89.9196, 6.5129) -> (-84.4965, -8.9388)
  spline S1373 degree 3 poles (-84.4965, -8.9388) (-84.1247, -9.9972) (-82.9079, -9.9705) (-82.9079, -10.3938) knots 0 0 0 0 1 1 1 1
  spline S1374 degree 3 poles (-82.9079, -10.3938) (-82.9079, -10.7115) (-83.1971, -11.267) (-83.4111, -11.267) knots 0 0 0 0 1 1 1 1
  spline S1375 degree 3 poles (-83.4111, -11.267) (-84.4664, -11.214) (-85.8448, -11.1903) (-87.2194, -11.1903) knots 0 0 0 0 1 1 1 1
  spline S1376 degree 3 poles (-87.2194, -11.1903) (-88.5939, -11.1903) (-89.9722, -11.214) (-91.0313, -11.267) knots 0 0 0 0 1 1 1 1
  spline S1377 degree 3 poles (-91.0313, -11.267) (-91.2416, -11.267) (-91.5045, -10.7115) (-91.5045, -10.3938) knots 0 0 0 0 1 1 1 1
  spline S1378 degree 3 poles (-91.5045, -10.3938) (-91.5045, -9.9705) (-89.8408, -9.9972) (-90.2088, -8.9388) knots 0 0 0 0 1 1 1 1
  line L306 (-90.2088, -8.9388) -> (-94.0996, 2.2533)
  spline S1379 degree 3 poles (-94.0996, 2.2533) (-95.3165, -1.2924) (-98.1219, -7.0866) (-97.6712, -8.9388) knots 0 0 0 0 1 1 1 1
  spline S1380 degree 3 poles (-97.6712, -8.9388) (-97.2994, -9.9972) (-96.1089, -9.9705) (-96.1089, -10.3938) knots 0 0 0 0 1 1 1 1
  spline S1381 degree 3 poles (-96.1089, -10.3938) (-96.1089, -10.7115) (-96.3755, -11.267) (-96.5859, -11.267) knots 0 0 0 0 1 1 1 1
  spline S1382 degree 3 poles (-96.5859, -11.267) (-97.645, -11.214) (-99.0195, -11.1903) (-100.3978, -11.1903) knots 0 0 0 0 1 1 1 1
  spline S1383 degree 3 poles (-100.3978, -11.1903) (-101.7987, -11.1903) (-103.1733, -11.214) (-104.206, -11.267) knots 0 0 0 0 1 1 1 1
  spline S1384 degree 3 poles (-104.206, -11.267) (-104.4163, -11.267) (-104.7093, -10.7115) (-104.7093, -10.3938) knots 0 0 0 0 1 1 1 1
  spline S1385 degree 3 poles (-104.7093, -10.3938) (-104.7093, -9.9705) (-103.0155, -9.9972) (-103.3873, -8.9122) knots 0 0 0 0 1 1 1 1
  line L307 (-103.3873, -8.9122) -> (-107.327, 2.4384)
  line L308 (-107.327, 2.4384) -> (-111.2704, -8.9122)
  spline S1386 degree 3 poles (-111.2704, -8.9122) (-111.6422, -9.9972) (-109.9747, -9.9705) (-109.9747, -10.3938) knots 0 0 0 0 1 1 1 1
  spline S1387 degree 3 poles (-109.9747, -10.3938) (-109.9747, -10.7115) (-110.2639, -11.2936) (-110.478, -11.267) knots 0 0 0 0 1 1 1 1
  spline S1388 degree 3 poles (-110.478, -11.267) (-110.8723, -11.214) (-111.6685, -11.1903) (-112.4609, -11.1903) knots 0 0 0 0 1 1 1 1
  spline S1389 degree 3 poles (-112.4609, -11.1903) (-113.2534, -11.1903) (-114.0496, -11.214) (-114.4439, -11.267) knots 0 0 0 0 1 1 1 1
  spline S1390 degree 3 poles (-114.4439, -11.267) (-114.688, -11.2936) (-114.9509, -10.7115) (-114.9509, -10.3938) knots 0 0 0 0 1 1 1 1
  spline S1391 degree 3 poles (-114.9509, -10.3938) (-114.9509, -9.9705) (-113.7604, -9.9972) (-113.3886, -8.9388) knots 0 0 0 0 1 1 1 1
  line L309 (-113.3886, -8.9388) -> (-107.9354, 6.5129)
  spline S1392 degree 3 poles (-107.9354, 6.5129) (-107.0378, 6.46) (-106.2717, 6.4337) (-105.5281, 6.4337) knots 0 0 0 0 1 1 1 1
  spline S1393 degree 3 poles (-105.5281, 6.4337) (-104.7619, 6.4337) (-104.0221, 6.46) (-103.0944, 6.5129) knots 0 0 0 0 1 1 1 1
  line L310 (-103.0944, 6.5129) -> (-99.0459, -5.0229)
  spline S1394 degree 3 poles (-99.0459, -5.0229) (-97.7765, -0.8688) (-95.2114, 3.9993) (-94.7607, 6.5129) knots 0 0 0 0 1 1 1 1
  line L311 (-94.7607, 6.5129) -> (-89.9196, 6.5129)
  spline S1395 degree 3 poles (151.9352, 6.2485) (151.9352, 10.5612) (153.8932, 12.5985) (157.7825, 12.5985) knots 0 0 0 0 1 1 1 1
  spline S1396 degree 3 poles (157.7825, 12.5985) (153.8932, 12.5985) (151.9352, 10.5612) (151.9352, 6.2485) knots -1 -1 -1 -1 0 0 0 0
  spline S1397 degree 3 poles (-159.8169, -9.362) (-155.8503, -9.362) (-154.4205, -6.1339) (-153.918, -6.1339) knots 0 0 0 0 1 1 1 1
  spline S1398 degree 3 poles (-153.918, -6.1339) (-154.4205, -6.1339) (-155.8503, -9.362) (-159.8169, -9.362) knots -1 -1 -1 -1 0 0 0 0
  line L312 (-159.9516, 3.7083) -> (-167.599, -8.9649)
  line L313 (-167.599, -8.9649) -> (-159.9516, 3.7083)
  line L314 (151.9352, -8.9386) -> (151.9352, 6.2485)
  spline S1399 degree 3 poles (151.9352, 6.2485) (151.9352, 10.5612) (153.8932, 12.5985) (157.7825, 12.5985) knots 0 0 0 0 1 1 1 1
  spline S1400 degree 3 poles (157.7825, 12.5985) (159.7669, 12.5985) (161.2221, 12.0958) (161.5661, 11.7518) knots 0 0 0 0 1 1 1 1
  spline S1401 degree 3 poles (161.5661, 11.7518) (161.7248, 11.5931) (161.3015, 10.6141) (161.0634, 10.6141) knots 0 0 0 0 1 1 1 1
  spline S1402 degree 3 poles (161.0634, 10.6141) (158.4175, 10.6141) (157.2798, 9.6881) (157.2798, 6.4866) knots 0 0 0 0 1 1 1 1
  line L315 (157.2798, 6.4866) -> (157.2798, -8.9386)
  spline S1403 degree 3 poles (157.2798, -8.9386) (157.2798, -10.0763) (158.7086, -9.9969) (158.7086, -10.3938) knots 0 0 0 0 1 1 1 1
  spline S1404 degree 3 poles (158.7086, -10.3938) (158.7086, -10.7113) (158.444, -11.2934) (158.2323, -11.2934) knots 0 0 0 0 1 1 1 1
  spline S1405 degree 3 poles (158.2323, -11.2934) (157.174, -11.2405) (155.8775, -11.214) (154.6075, -11.214) knots 0 0 0 0 1 1 1 1
  spline S1406 degree 3 poles (154.6075, -11.214) (153.3111, -11.214) (152.012, -11.2405) (150.9827, -11.2934) knots 0 0 0 0 1 1 1 1
  spline S1407 degree 3 poles (150.9827, -11.2934) (150.7684, -11.2934) (150.48, -10.7113) (150.48, -10.3938) knots 0 0 0 0 1 1 1 1
  spline S1408 degree 3 poles (150.48, -10.3938) (150.48, -9.9969) (151.9352, -10.0763) (151.9352, -8.9386) knots 0 0 0 0 1 1 1 1
  line L316 (-84.4965, -8.9388) -> (-89.9196, 6.5129)
  line L317 (-89.9196, 6.5129) -> (-84.4965, -8.9388)
  spline S1409 degree 3 poles (-152.7783, 5.6398) (-152.7783, 5.2166) (-152.8314, 5.1373) (-153.4155, 4.1847) knots 0 0 0 0 1 1 1 1
  spline S1410 degree 3 poles (-153.4155, 4.1847) (-152.8314, 5.1373) (-152.7783, 5.2166) (-152.7783, 5.6398) knots -1 -1 -1 -1 0 0 0 0
  line L318 (151.9352, 6.2485) -> (151.9352, -8.9386)
  line L319 (151.9352, -8.9386) -> (151.9352, 6.2485)
  spline S1411 degree 3 poles (265.5433, 3.7879) (268.7186, 3.7879) (270.6236, 1.195) (270.6236, -3.303) knots -1 -1 -1 -1 0 0 0 0
  spline S1412 degree 3 poles (270.6236, -3.303) (270.6236, -7.2717) (269.1417, -9.653) (266.6546, -9.653) knots -1 -1 -1 -1 0 0 0 0
  spline S1413 degree 3 poles (266.6546, -9.653) (263.4529, -9.653) (262.1297, -5.7371) (261.6537, -5.7371) knots -1 -1 -1 -1 0 0 0 0
  spline S1414 degree 3 poles (261.6537, -5.7371) (261.336, -5.7371) (260.7539, -6.2928) (260.7539, -6.5044) knots -1 -1 -1 -1 0 0 0 0
  spline S1415 degree 3 poles (260.7539, -6.5044) (260.7539, -6.7161) (261.336, -10.0763) (261.442, -10.4732) knots -1 -1 -1 -1 0 0 0 0
  spline S1416 degree 3 poles (261.442, -10.4732) (261.5743, -10.9759) (261.786, -11.2934) (262.1297, -11.2934) knots -1 -1 -1 -1 0 0 0 0
  spline S1417 degree 3 poles (262.1297, -11.2934) (262.5533, -11.2934) (262.765, -11.0288) (263.4264, -11.0288) knots -1 -1 -1 -1 0 0 0 0
  spline S1418 degree 3 poles (263.4264, -11.0288) (264.326, -11.0288) (265.305, -11.558) (267.4219, -11.558) knots -1 -1 -1 -1 0 0 0 0
  spline S1419 degree 3 poles (267.4219, -11.558) (272.6876, -11.558) (276.4447, -7.748) (276.4447, -2.3769) knots -1 -1 -1 -1 0 0 0 0
  spline S1420 degree 3 poles (276.4447, -2.3769) (276.4447, 2.9412) (272.767, 6.7777) (267.66, 6.7777) knots -1 -1 -1 -1 0 0 0 0
  spline S1421 degree 3 poles (267.66, 6.7777) (262.2093, 6.7777) (259.9339, 2.412) (259.9339, 1.5389) knots -1 -1 -1 -1 0 0 0 0
  spline S1422 degree 3 poles (259.9339, 1.5389) (259.9339, 1.3272) (260.7277, 1.0891) (260.8862, 1.2743) knots -1 -1 -1 -1 0 0 0 0
  spline S1423 degree 3 poles (260.8862, 1.2743) (262.4475, 3.0206) (263.8233, 3.7879) (265.5433, 3.7879) knots -1 -1 -1 -1 0 0 0 0
  spline S1424 degree 3 poles (262.1297, -11.2934) (261.786, -11.2934) (261.5743, -10.9759) (261.442, -10.4732) knots 0 0 0 0 1 1 1 1
  spline S1425 degree 3 poles (261.442, -10.4732) (261.5743, -10.9759) (261.786, -11.2934) (262.1297, -11.2934) knots -1 -1 -1 -1 0 0 0 0
  spline S1426 degree 3 poles (260.8862, 1.2743) (260.7277, 1.0891) (259.9339, 1.3272) (259.9339, 1.5389) knots 0 0 0 0 1 1 1 1
  spline S1427 degree 3 poles (259.9339, 1.5389) (259.9339, 1.3272) (260.7277, 1.0891) (260.8862, 1.2743) knots -1 -1 -1 -1 0 0 0 0
  spline S1428 degree 3 poles (261.442, -10.4732) (261.336, -10.0763) (260.7539, -6.7161) (260.7539, -6.5044) knots 0 0 0 0 1 1 1 1
  spline S1429 degree 3 poles (260.7539, -6.5044) (260.7539, -6.7161) (261.336, -10.0763) (261.442, -10.4732) knots -1 -1 -1 -1 0 0 0 0
  spline S1430 degree 3 poles (259.9339, 1.5389) (259.9339, 2.412) (262.2093, 6.7777) (267.66, 6.7777) knots 0 0 0 0 1 1 1 1
  spline S1431 degree 3 poles (267.66, 6.7777) (262.2093, 6.7777) (259.9339, 2.412) (259.9339, 1.5389) knots -1 -1 -1 -1 0 0 0 0
  spline S1432 degree 3 poles (260.7539, -6.5044) (260.7539, -6.2928) (261.336, -5.7371) (261.6537, -5.7371) knots 0 0 0 0 1 1 1 1
  spline S1433 degree 3 poles (261.6537, -5.7371) (261.336, -5.7371) (260.7539, -6.2928) (260.7539, -6.5044) knots -1 -1 -1 -1 0 0 0 0
  spline S1434 degree 3 poles (267.66, 6.7777) (272.767, 6.7777) (276.4447, 2.9412) (276.4447, -2.3769) knots 0 0 0 0 1 1 1 1
  spline S1435 degree 3 poles (276.4447, -2.3769) (276.4447, 2.9412) (272.767, 6.7777) (267.66, 6.7777) knots -1 -1 -1 -1 0 0 0 0
  spline S1436 degree 3 poles (-107.9354, 6.5129) (-107.0378, 6.46) (-106.2717, 6.4337) (-105.5281, 6.4337) knots 0 0 0 0 1 1 1 1
  spline S1437 degree 3 poles (-105.5281, 6.4337) (-106.2717, 6.4337) (-107.0378, 6.46) (-107.9354, 6.5129) knots -1 -1 -1 -1 0 0 0 0
  spline S1438 degree 3 poles (-160.1069, 6.4339) (-157.6232, 6.4339) (-155.1354, 6.4601) (-153.2807, 6.5132) knots 0 0 0 0 1 1 1 1
  spline S1439 degree 3 poles (-153.2807, 6.5132) (-155.1354, 6.4601) (-157.6232, 6.4339) (-160.1069, 6.4339) knots -1 -1 -1 -1 0 0 0 0
  spline S1440 degree 3 poles (158.2323, -11.2934) (157.174, -11.2405) (155.8775, -11.214) (154.6075, -11.214) knots 0 0 0 0 1 1 1 1
  spline S1441 degree 3 poles (154.6075, -11.214) (155.8775, -11.214) (157.174, -11.2405) (158.2323, -11.2934) knots -1 -1 -1 -1 0 0 0 0
  spline S1442 degree 3 poles (161.5661, 11.7518) (161.7248, 11.5931) (161.3015, 10.6141) (161.0634, 10.6141) knots 0 0 0 0 1 1 1 1
  spline S1443 degree 3 poles (161.0634, 10.6141) (161.3015, 10.6141) (161.7248, 11.5931) (161.5661, 11.7518) knots -1 -1 -1 -1 0 0 0 0
  spline S1444 degree 3 poles (-167.7828, 1.486) (-168.1014, 1.486) (-168.657, 1.7508) (-168.657, 1.9624) knots 0 0 0 0 1 1 1 1
  spline S1445 degree 3 poles (-168.657, 1.9624) (-168.657, 1.7508) (-168.1014, 1.486) (-167.7828, 1.486) knots -1 -1 -1 -1 0 0 0 0
  spline S1446 degree 3 poles (-94.0996, 2.2533) (-95.3165, -1.2924) (-98.1219, -7.0866) (-97.6712, -8.9388) knots 0 0 0 0 1 1 1 1
  spline S1447 degree 3 poles (-97.6712, -8.9388) (-98.1219, -7.0866) (-95.3165, -1.2924) (-94.0996, 2.2533) knots -1 -1 -1 -1 0 0 0 0
  spline S1448 degree 3 poles (82.8525, 6.5131) (83.2494, 6.4602) (84.0167, 6.4337) (84.784, 6.4337) knots 0 0 0 0 1 1 1 1
  spline S1449 degree 3 poles (84.784, 6.4337) (84.0167, 6.4337) (83.2494, 6.4602) (82.8525, 6.5131) knots -1 -1 -1 -1 0 0 0 0
  spline S1450 degree 3 poles (87.2182, -10.3673) (87.2182, -10.6848) (86.9536, -11.3225) (86.7419, -11.2934) knots 0 0 0 0 1 1 1 1
  spline S1451 degree 3 poles (86.7419, -11.2934) (86.9536, -11.3225) (87.2182, -10.6848) (87.2182, -10.3673) knots -1 -1 -1 -1 0 0 0 0
  spline S1452 degree 3 poles (-110.478, -11.267) (-110.8723, -11.214) (-111.6685, -11.1903) (-112.4609, -11.1903) knots 0 0 0 0 1 1 1 1
  spline S1453 degree 3 poles (-112.4609, -11.1903) (-111.6685, -11.1903) (-110.8723, -11.214) (-110.478, -11.267) knots -1 -1 -1 -1 0 0 0 0
  spline S1454 degree 3 poles (84.784, 6.4337) (85.5513, 6.4337) (86.3186, 6.4602) (86.7419, 6.5131) knots 0 0 0 0 1 1 1 1
  spline S1455 degree 3 poles (86.7419, 6.5131) (86.3186, 6.4602) (85.5513, 6.4337) (84.784, 6.4337) knots -1 -1 -1 -1 0 0 0 0
  spline S1456 degree 3 poles (85.9217, -8.9121) (85.9217, -10.0498) (87.2182, -9.9705) (87.2182, -10.3673) knots 0 0 0 0 1 1 1 1
  spline S1457 degree 3 poles (87.2182, -10.3673) (87.2182, -9.9705) (85.9217, -10.0498) (85.9217, -8.9121) knots -1 -1 -1 -1 0 0 0 0
  spline S1458 degree 3 poles (-97.6712, -8.9388) (-97.2994, -9.9972) (-96.1089, -9.9705) (-96.1089, -10.3938) knots 0 0 0 0 1 1 1 1
  spline S1459 degree 3 poles (-96.1089, -10.3938) (-96.1089, -9.9705) (-97.2994, -9.9972) (-97.6712, -8.9388) knots -1 -1 -1 -1 0 0 0 0
  spline S1460 degree 3 poles (86.7419, 6.5131) (86.9536, 6.5395) (87.2182, 5.9575) (87.2182, 5.64) knots 0 0 0 0 1 1 1 1
  spline S1461 degree 3 poles (87.2182, 5.64) (87.2182, 5.9575) (86.9536, 6.5395) (86.7419, 6.5131) knots -1 -1 -1 -1 0 0 0 0
  line L320 (85.9217, -8.9121) -> (85.9217, 4.1583)
  line L321 (85.9217, 4.1583) -> (85.9217, -8.9121)
  spline S1462 degree 3 poles (-109.9747, -10.3938) (-109.9747, -10.7115) (-110.2639, -11.2936) (-110.478, -11.267) knots 0 0 0 0 1 1 1 1
  spline S1463 degree 3 poles (-110.478, -11.267) (-110.2639, -11.2936) (-109.9747, -10.7115) (-109.9747, -10.3938) knots -1 -1 -1 -1 0 0 0 0
  spline S1464 degree 3 poles (69.4117, -10.3938) (69.4117, -9.9705) (70.7082, -10.0498) (70.7082, -8.9121) knots 0 0 0 0 1 1 1 1
  spline S1465 degree 3 poles (70.7082, -8.9121) (70.7082, -10.0498) (69.4117, -9.9705) (69.4117, -10.3938) knots -1 -1 -1 -1 0 0 0 0
  spline S1466 degree 3 poles (-96.1089, -10.3938) (-96.1089, -10.7115) (-96.3755, -11.267) (-96.5859, -11.267) knots 0 0 0 0 1 1 1 1
  spline S1467 degree 3 poles (-96.5859, -11.267) (-96.3755, -11.267) (-96.1089, -10.7115) (-96.1089, -10.3938) knots -1 -1 -1 -1 0 0 0 0
  spline S1468 degree 3 poles (138.5209, 6.5131) (138.7325, 6.5131) (139.0236, 5.9575) (139.0236, 5.64) knots 0 0 0 0 1 1 1 1
  spline S1469 degree 3 poles (139.0236, 5.64) (139.0236, 5.9575) (138.7325, 6.5131) (138.5209, 6.5131) knots -1 -1 -1 -1 0 0 0 0
  spline S1470 degree 3 poles (-111.2704, -8.9122) (-111.6422, -9.9972) (-109.9747, -9.9705) (-109.9747, -10.3938) knots 0 0 0 0 1 1 1 1
  spline S1471 degree 3 poles (-109.9747, -10.3938) (-109.9747, -9.9705) (-111.6422, -9.9972) (-111.2704, -8.9122) knots -1 -1 -1 -1 0 0 0 0
  spline S1472 degree 3 poles (-96.5859, -11.267) (-97.645, -11.214) (-99.0195, -11.1903) (-100.3978, -11.1903) knots 0 0 0 0 1 1 1 1
  spline S1473 degree 3 poles (-100.3978, -11.1903) (-99.0195, -11.1903) (-97.645, -11.214) (-96.5859, -11.267) knots -1 -1 -1 -1 0 0 0 0
  spline S1474 degree 3 poles (145.2942, -11.214) (143.9977, -11.214) (142.7013, -11.2405) (141.6694, -11.2934) knots 0 0 0 0 1 1 1 1
  spline S1475 degree 3 poles (141.6694, -11.2934) (142.7013, -11.2405) (143.9977, -11.214) (145.2942, -11.214) knots -1 -1 -1 -1 0 0 0 0
  line L322 (-111.2704, -8.9122) -> (-107.327, 2.4384)
  line L323 (-107.327, 2.4384) -> (-111.2704, -8.9122)
  spline S1476 degree 3 poles (-100.3978, -11.1903) (-101.7987, -11.1903) (-103.1733, -11.214) (-104.206, -11.267) knots 0 0 0 0 1 1 1 1
  spline S1477 degree 3 poles (-104.206, -11.267) (-103.1733, -11.214) (-101.7987, -11.1903) (-100.3978, -11.1903) knots -1 -1 -1 -1 0 0 0 0
  line L324 (142.6219, -2.7209) -> (142.6219, -8.965)
  line L325 (142.6219, -8.965) -> (142.6219, -2.7209)
  line L326 (-107.327, 2.4384) -> (-103.3873, -8.9122)
  line L327 (-103.3873, -8.9122) -> (-107.327, 2.4384)
  spline S1478 degree 3 poles (-104.206, -11.267) (-104.4163, -11.267) (-104.7093, -10.7115) (-104.7093, -10.3938) knots 0 0 0 0 1 1 1 1
  spline S1479 degree 3 poles (-104.7093, -10.3938) (-104.7093, -10.7115) (-104.4163, -11.267) (-104.206, -11.267) knots -1 -1 -1 -1 0 0 0 0
  line L328 (-89.9196, 6.5129) -> (-94.7607, 6.5129)
  line L329 (-94.7607, 6.5129) -> (-89.9196, 6.5129)
  spline S1480 degree 3 poles (141.1667, -10.4203) (141.1667, -10.0234) (142.6219, -10.1028) (142.6219, -8.965) knots 0 0 0 0 1 1 1 1
  line L330 (142.6219, -8.965) -> (142.6219, -2.7209)
  line L331 (142.6219, -2.7209) -> (136.1661, -8.8857)
  spline S1481 degree 3 poles (136.1661, -8.8857) (135.3723, -9.6794) (137.1715, -9.9705) (137.1715, -10.3938) knots 0 0 0 0 1 1 1 1
  spline S1482 degree 3 poles (137.1715, -10.3938) (137.1715, -10.7113) (136.8011, -11.2934) (136.5894, -11.2669) knots 0 0 0 0 1 1 1 1
  spline S1483 degree 3 poles (136.5894, -11.2669) (136.0602, -11.214) (135.0284, -11.1902) (133.9965, -11.1902) knots 0 0 0 0 1 1 1 1
  spline S1484 degree 3 poles (133.9965, -11.1902) (132.9884, -11.1902) (131.9592, -11.214) (131.4274, -11.2669) knots 0 0 0 0 1 1 1 1
  spline S1485 degree 3 poles (131.4274, -11.2669) (131.2157, -11.2934) (130.9247, -10.7113) (130.9247, -10.3938) knots 0 0 0 0 1 1 1 1